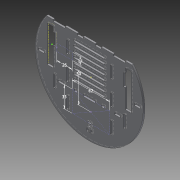
# Autodesk Inventor part: Base Plate
Saved by Autodesk Inventor 2015 (Build 190159000, 159)
## iProperties
Created: 2014-11-10
Part Number: Base Plate
Material: Generic
Document SubType Name: Modeling
Designer: karl
Density: 1 g/cm^3
Appearance: Default
Author: karl
Autodesk Inventor part; units mm, degrees
ref_plane "YZ Plane" through (0, 0, 0) normal (1, 0, 0) x (0, 1, 0)
ref_plane "XZ Plane" through (0, 0, 0) normal (0, 1, 0) x (-1, 0, 0)
ref_plane "XY Plane" through (0, 0, 0) normal (0, 0, 1) x (1, 0, 0)
sketch "Sketch1" plane through (0, 0, 0) normal (0, 1, 0) x (-1, 0, 0)
  circle A0 centre (0, 0) radius 90
  line L0 (-71.239, 55) -> (71.239, 55)
  dimension "d0" = 180
  dimension "d1" = 55
  constraints: 2 end point, 2 point on circle, 1 centre point, 1 coincident, 1 horizontal
  measures "d0" diameter of A0
  measures "d1" distance from line of point (0, 0) L0
extrude "Extrusion1" add sketch "Sketch1" along normal blind 3 contours A0 L0 picked at (-1.0947, 6.6866)
sketch "Sketch2" plane through (0, 3, 0) normal (0, 1, 0) x (1, 0, 0)
  line L0 (-70, -45) -> (-60, -45)
  line L1 (-60, -45) -> (-60, 15)
  line L2 (-60, 15) -> (-70, 15)
  line L3 (-70, 15) -> (-70, -45)
  line L4 (-70, -45) -> (-60, 15) construction
  line L5 (-60, -45) -> (-70, 15) construction
  point P0 (0, 0)
  point P1 (-65, -15)
  dimension "d4" = 10
  dimension "d5" = 60
  dimension "d6" = 15
  dimension "d7" = 65
  constraints: 12 end point, 2 midpoint, 2 parallel, 1 horizontal, 1 perpendicular
  measures "d4" distance of L2.end L1.end
  measures "d5" distance of L1.end L0.end
  measures "d6" vertical distance of point (0, 0) point (-65, -15)
  measures "d7" horizontal distance of point (0, 0) point (-65, -15)
extrude "Extrusion2" cut sketch "Sketch2" against normal blind 3
sketch "Sketch3" plane through (0, 3, 0) normal (0, 1, 0) x (1, 0, 0)
  line L0 (-71.239, -55) -> (71.239, -55) projected
  line L1 (-60, -55) -> (-40, -55)
  line L2 (-40, -55) -> (-40, -52)
  line L3 (-40, -52) -> (-60, -52)
  line L4 (-60, -52) -> (-60, -55)
  line L5 (-20, -55) -> (-10, -55)
  line L6 (-10, -55) -> (-10, -52)
  line L7 (-10, -52) -> (-20, -52)
  line L8 (-20, -52) -> (-20, -55)
  point P0 (0, 0)
  dimension "d10" = 20
  dimension "d11" = 3
  dimension "d12" = 10
  dimension "d13" = 3
  dimension "d14" = 10
  dimension "d15" = 20
  constraints: 16 end point, 4 parallel, 2 horizontal, 2 perpendicular, 2 point on line
  measures "d10" distance of L3.end L2.end
  measures "d11" distance of L2.end L1.end
  measures "d12" distance of L7.end L6.end
  measures "d13" distance of L6.end L5.end
  measures "d14" distance from line of point (0, 0) L6
  measures "d15" distance between parallel lines of L8 L2
extrude "Extrusion3" cut sketch "Sketch3" against normal blind 3
sketch "Sketch4" plane through (0, 3, 0) normal (0, 1, 0) x (1, 0, 0)
  line L0 (-60, -45) -> (-60, 15) projected
  line L1 (-60, -37) -> (-57, -37)
  line L2 (-57, -37) -> (-57, -17)
  line L3 (-57, -17) -> (-60, -17)
  line L4 (-60, -17) -> (-60, -37)
  line L5 (-57, 43) -> (-60, 43)
  line L6 (-60, 43) -> (-60, 23)
  line L7 (-60, 23) -> (-57, 23)
  line L8 (-57, 23) -> (-57, 43)
  line L9 (-60, -52) -> (-40, -52) projected
  point P0 (0, 0)
  dimension "d18" = 3
  dimension "d19" = 20
  dimension "d20" = 3
  dimension "d21" = 20
  dimension "d22" = 40
  dimension "d23" = 15
  constraints: 16 end point, 4 parallel, 2 horizontal, 2 perpendicular, 2 point on line
  measures "d18" distance of L3.end L2.end
  measures "d19" distance of L2.end L1.end
  measures "d20" distance of L7.end L6.end
  measures "d21" distance of L6.end L5.end
  measures "d22" distance between parallel lines of L3 L7
  measures "d23" distance between parallel lines of L9 L1
extrude "Extrusion4" cut sketch "Sketch4" against normal blind 3
sketch "Sketch5" plane through (0, 3, 0) normal (0, 1, 0) x (1, 0, 0)
  line L0 (31, 67.5) -> (-31, 67.5) construction
  line L1 (-31, 67.5) -> (-31, 32.5) construction
  line L2 (-31, 32.5) -> (31, 32.5) construction
  line L3 (31, 32.5) -> (31, 67.5) construction
  line L4 (31, 67.5) -> (-31, 32.5) construction
  line L5 (-31, 67.5) -> (31, 32.5) construction
  line L6 (-57, -37) -> (-57, -17) construction
  line L7 (-57, -21) -> (-31, -21) construction
  line L8 (-31, -21) -> (-31, -9) construction
  line L9 (-31, -9) -> (-57, -9) construction
  line L10 (-57, -9) -> (-57, -21) construction
  line L11 (-60, -45) -> (-70, -45) construction
  line L12 (-70, -45) -> (-70, 15) construction
  line L13 (-70, -15) -> (-60, -15) construction
  point P0 (0, 0)
  point P1 (0, 50)
  point P2 (0, 50)
  point P3 (-57, -15)
  point P4 (-65, -15)
  dimension "d26" = 62
  dimension "d27" = 35
  dimension "d28" = 50
  dimension "d29" = 26
  dimension "d30" = 12
  constraints: 22 end point, 6 midpoint, 4 parallel, 3 horizontal, 2 perpendicular, 1 horizontal alignment, 1 point on line, 1 vertical alignment
  measures "d26" distance of L2.end L1.end
  measures "d27" distance of L1.end L0.end
  measures "d28" distance of point (0, 0) point (0, 50)
  measures "d29" distance of L9.end L8.end
  measures "d30" distance of L8.end L7.end
sketch "Sketch6" plane through (0, 3, 0) normal (0, 1, 0) x (1, 0, 0)
  line L0 (-38, 63) -> (-35, 63)
  line L1 (-35, 63) -> (-35, 43)
  line L2 (-35, 43) -> (-38, 43)
  line L3 (-38, 43) -> (-38, 63)
  line L4 (-38, 3) -> (-35, 3)
  line L5 (-35, 3) -> (-35, 23)
  line L6 (-35, 23) -> (-38, 23)
  line L7 (-38, 23) -> (-38, 3)
  line L8 (-38, -37) -> (-35, -37)
  line L9 (-35, -37) -> (-35, -17)
  line L10 (-35, -17) -> (-38, -17)
  line L11 (-38, -17) -> (-38, -37)
  line L12 (-60, -52) -> (-40, -52) projected
  point P0 (0, 0)
  dimension "d32" = 3
  dimension "d33" = 20
  dimension "d34" = 35
  dimension "d35" = 3
  dimension "d36" = 20
  dimension "d37" = 20
  dimension "d38" = 3
  dimension "d39" = 20
  dimension "d40" = 20
  dimension "d41" = 15
  constraints: 24 end point, 6 parallel, 3 horizontal, 3 perpendicular, 2 collinear
  measures "d32" distance of L1.end L2.end
  measures "d33" distance of L0.end L1.end
  measures "d34" distance from line of point (0, 0) L1
  measures "d35" distance of L6.end L5.end
  measures "d36" distance of L5.end L4.end
  measures "d37" distance between parallel lines of L2 L6
  measures "d38" distance of L10.end L9.end
  measures "d39" distance of L9.end L8.end
  measures "d40" distance between parallel lines of L4 L10
  measures "d41" distance between parallel lines of L8 L12
extrude "Extrusion5" cut sketch "Sketch6" against normal blind 3
sketch "Sketch7" plane through (0, 3, 0) normal (0, 1, 0) x (1, 0, 0)
  line L0 (-10, 31) -> (10, 31)
  line L1 (10, 31) -> (10, 28)
  line L2 (10, 28) -> (-10, 28)
  line L3 (-10, 28) -> (-10, 31)
  line L4 (-60, -52) -> (-40, -52) projected
  line L5 (-20, 28) -> (-25, 28)
  line L6 (-25, 28) -> (-25, 31)
  line L7 (-25, 31) -> (-20, 31)
  line L8 (-20, 31) -> (-20, 28)
  line L9 (-42, 28) -> (-52, 28)
  line L10 (-52, 28) -> (-52, 31)
  line L11 (-52, 31) -> (-42, 31)
  line L12 (-42, 31) -> (-42, 28)
  point P0 (0, 0)
  point P1 (0, 28)
  dimension "d44" = 20
  dimension "d45" = 3
  dimension "d46" = 80
  dimension "d47" = 5
  dimension "d48" = 3
  dimension "d49" = 10
  dimension "d58" = 10
  dimension "d59" = 3
  dimension "d60" = 17
  constraints: 24 end point, 6 parallel, 3 horizontal, 3 perpendicular, 2 collinear, 1 midpoint, 1 vertical alignment
  measures "d44" distance of L1.end L2.end
  measures "d45" distance of L0.end L1.end
  measures "d46" distance between parallel lines of L4 L2
  measures "d47" distance of L6.end L7.end
  measures "d48" distance of L5.end L6.end
  measures "d49" distance between parallel lines of L3 L8
  measures "d58" distance of L10.end L11.end
  measures "d59" distance of L9.end L10.end
  measures "d60" distance between parallel lines of L6 L12
extrude "Extrusion6" cut sketch "Sketch7" against normal blind 3
sketch "Sketch8" plane through (0, 3, 0) normal (0, 1, 0) x (1, 0, 0)
  line L0 (-4.5, 73) -> (-1.5, 73)
  line L1 (-1.5, 73) -> (-1.5, 78)
  line L2 (-1.5, 78) -> (-4.5, 78)
  line L3 (-4.5, 78) -> (-4.5, 73)
  line L4 (-10, 31) -> (10, 31) projected
  point P0 (0, 0)
  dimension "d52" = 3
  dimension "d53" = 5
  dimension "d54" = 1.5
  dimension "d55" = 42
  constraints: 8 end point, 2 parallel, 1 horizontal, 1 perpendicular
  measures "d52" distance of L2.end L1.end
  measures "d53" distance of L1.end L0.end
  measures "d54" distance from line of L1 point (0, 0)
  measures "d55" distance between parallel lines of L4 L0
extrude "Extrusion7" cut sketch "Sketch8" against normal blind 3
mirror "Mirror1" about plane through (0, 0, 0) normal (1, 0, 0) of "Extrusion2", "Extrusion3", "Extrusion4", "Extrusion5", "Extrusion6", "Extrusion7"
sketch "Sketch9" plane through (0, 3, 0) normal (0, 1, 0) x (1, 0, 0)
  line L0 (75, -1.5) -> (85, -1.5)
  line L1 (85, -1.5) -> (85, 1.5)
  line L2 (85, 1.5) -> (75, 1.5)
  line L3 (75, 1.5) -> (75, -1.5)
  line L4 (70, -45) -> (70, 15) projected
  point P0 (0, 0)
  point P1 (75, 0)
  dimension "d61" = 10
  dimension "d62" = 3
  dimension "d63" = 5
  constraints: 8 end point, 2 parallel, 1 horizontal, 1 horizontal alignment, 1 midpoint, 1 perpendicular
  measures "d61" distance of L2.end L1.end
  measures "d62" distance of L1.end L0.end
  measures "d63" distance between parallel lines of L4 L3
extrude "Extrusion8" cut sketch "Sketch9" against normal blind 3
mirror "Mirror2" about plane through (0, 0, 0) normal (1, 0, 0) of "Extrusion8"
sketch "Sketch10" plane through (0, 3, 0) normal (0, 1, 0) x (1, 0, 0)
  line L0 (2.5, 64) -> (-2.5, 64) construction
  line L1 (2.5, 65) -> (-2.5, 65)
  line L2 (-2.5, 63) -> (2.5, 63)
  arc A0 (2.5, 63) -> (2.5, 65) centre (2.5, 64) ccw
  arc A1 (-2.5, 65) -> (-2.5, 63) centre (-2.5, 64) ccw
  line L3 (2.5, 69) -> (-2.5, 69) construction
  line L4 (2.5, 70) -> (-2.5, 70)
  line L5 (-2.5, 68) -> (2.5, 68)
  arc A2 (2.5, 68) -> (2.5, 70) centre (2.5, 69) ccw
  arc A3 (-2.5, 70) -> (-2.5, 68) centre (-2.5, 69) ccw
  point P0 (0, 0)
  point P1 (0, 64)
  point P2 (0, 69)
  dimension "d66" = 2
  dimension "d67" = 2
  dimension "d68" = 3
  dimension "d69" = 63
  dimension "d70" = 5
  constraints: 16 end point, 8 point on circle, 8 tangent, 4 centre point, 3 parallel, 3 vertical alignment, 2 midpoint, 1 horizontal
  measures "d66" diameter of A1
  measures "d67" diameter of A3
  measures "d68" distance between parallel lines of L1 L5
  measures "d69" distance from line of point (0, 0) L2
  measures "d70" distance of L0.start L0.end
extrude "Extrusion9" cut sketch "Sketch10" against normal blind 3
sketch "Sketch11" plane through (0, 3, 0) normal (0, 1, 0) x (1, 0, 0)
  line L0 (25, -42) -> (-25, -42) construction
  line L1 (25, -40.5) -> (-25, -40.5)
  line L2 (-25, -43.5) -> (25, -43.5)
  arc A0 (25, -43.5) -> (25, -40.5) centre (25, -42) ccw
  arc A1 (-25, -40.5) -> (-25, -43.5) centre (-25, -42) ccw
  line L3 (0, -43.5) -> (0, -40.5) construction
  line L4 (25, -34) -> (-25, -34) construction
  line L5 (25, -32.5) -> (-25, -32.5)
  line L6 (-25, -35.5) -> (25, -35.5)
  arc A2 (25, -35.5) -> (25, -32.5) centre (25, -34) ccw
  arc A3 (-25, -32.5) -> (-25, -35.5) centre (-25, -34) ccw
  line L7 (0, -35.5) -> (0, -32.5) construction
  line L8 (25, -26) -> (-25, -26) construction
  line L9 (25, -24.5) -> (-25, -24.5)
  line L10 (-25, -27.5) -> (25, -27.5)
  arc A4 (25, -27.5) -> (25, -24.5) centre (25, -26) ccw
  arc A5 (-25, -24.5) -> (-25, -27.5) centre (-25, -26) ccw
  line L11 (0, -27.5) -> (0, -24.5) construction
  line L12 (25, -18) -> (-25, -18) construction
  line L13 (25, -16.5) -> (-25, -16.5)
  line L14 (-25, -19.5) -> (25, -19.5)
  arc A6 (25, -19.5) -> (25, -16.5) centre (25, -18) ccw
  arc A7 (-25, -16.5) -> (-25, -19.5) centre (-25, -18) ccw
  line L15 (0, -19.5) -> (0, -16.5) construction
  line L16 (25, -10) -> (-25, -10) construction
  line L17 (25, -8.5) -> (-25, -8.5)
  line L18 (-25, -11.5) -> (25, -11.5)
  arc A8 (25, -11.5) -> (25, -8.5) centre (25, -10) ccw
  arc A9 (-25, -8.5) -> (-25, -11.5) centre (-25, -10) ccw
  line L19 (0, -11.5) -> (0, -8.5) construction
  line L20 (25, -2) -> (-25, -2) construction
  line L21 (25, -0.5) -> (-25, -0.5)
  line L22 (-25, -3.5) -> (25, -3.5)
  arc A10 (25, -3.5) -> (25, -0.5) centre (25, -2) ccw
  arc A11 (-25, -0.5) -> (-25, -3.5) centre (-25, -2) ccw
  line L23 (0, -3.5) -> (0, -0.5) construction
  line L24 (25, 6) -> (-25, 6) construction
  line L25 (25, 7.5) -> (-25, 7.5)
  line L26 (-25, 4.5) -> (25, 4.5)
  arc A12 (25, 4.5) -> (25, 7.5) centre (25, 6) ccw
  arc A13 (-25, 7.5) -> (-25, 4.5) centre (-25, 6) ccw
  line L27 (0, 4.5) -> (0, 7.5) construction
  line L28 (25, 14) -> (-25, 14) construction
  line L29 (25, 15.5) -> (-25, 15.5)
  line L30 (-25, 12.5) -> (25, 12.5)
  arc A14 (25, 12.5) -> (25, 15.5) centre (25, 14) ccw
  arc A15 (-25, 15.5) -> (-25, 12.5) centre (-25, 14) ccw
  line L31 (0, 12.5) -> (0, 15.5) construction
  line L32 (10, -52) -> (20, -52) construction
  point P0 (0, 0)
  point P1 (0, -42)
  point P2 (0, -34)
  point P3 (0, -26)
  point P4 (0, -18)
  point P5 (0, -10)
  point P6 (0, -2)
  point P7 (0, 6)
  point P8 (0, 14)
  point P9 (0, -42)
  dimension "d73" = 3
  dimension "d74" = 50
  dimension "d77" = 8
  dimension "d82" = 10
  constraints: 80 end point, 32 point on circle, 16 centre point, 4 midpoint, 4 tangent, 2 vertical alignment, 1 collinear, 1 horizontal, 1 parallel, 1 vertical, 104 other
  measures "d73" diameter of A1
  measures "d74" distance of L0.start L0.end
  measures "d77" distance of L1.start L5.start
  measures "d82" distance between parallel lines of L32 L0
extrude "Extrusion10" cut sketch "Sketch11" against normal blind 3
equation "\"d40\" = d36"
body "Solid1"
